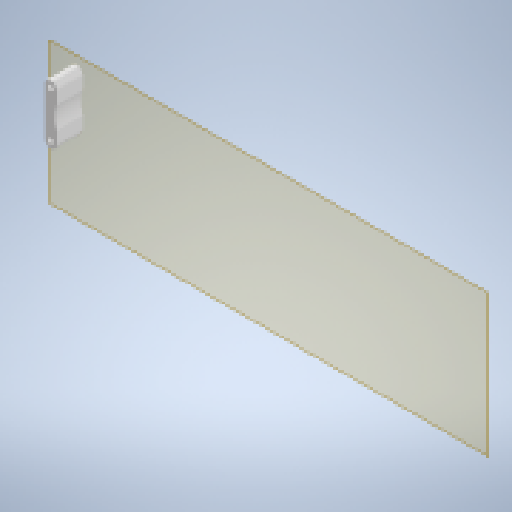
# Autodesk Inventor part: plate_washer_1
Saved by Autodesk Inventor 2024 (Build 280153000, 153)
## iProperties
Created: 2026-02-04
Part Number: plate_washer_1
Material: Generic
Document SubType Name: Modeling
Designer: SEMEN
Density: 1 g/cm^3
Appearance: Default
Author: SEMEN
Autodesk Inventor part; units mm, degrees
ref_plane "YZ Plane" through (0, 0, 0) normal (1, 0, 0) x (0, 1, 0)
ref_plane "XZ Plane" through (0, 0, 0) normal (0, 1, 0) x (-1, 0, 0)
ref_plane "XY Plane" through (0, 0, 0) normal (0, 0, 1) x (1, 0, 0)
ref_plane "Work Plane1" through (0, 0, 0) normal (0, 0, 1) x (1, 0, 0)
sketch "Sketch1" plane through (0, 0, 0) normal (0, 0, 1) x (1, 0, 0)
  circle A0 centre (-26, -15.5) radius 1.7 projected
  circle A1 centre (-26, 15.5) radius 1.7 projected
  arc A2 (-30.2, -15.5) -> (-21.8, -15.5) centre (-26, -15.5) ccw
  arc A3 (-21.8, 15.5) -> (-30.2, 15.5) centre (-26, 15.5) ccw
  arc A4 (-21.8, 7.3321) -> (-21.8, -7.3321) centre (0, 0) ccw
  line L0 (-21.8, -15.5) -> (-21.8, -7.3321)
  line L1 (-21.8, 7.3321) -> (-21.8, 15.5)
  line L2 (-30.2, -15.5) -> (-30.2, 15.5)
  line L3 (-26, -15.5) -> (-30.2, -15.5) construction
  dimension "d0" = 2.5
  dimension "d1" = 2.5
  dimension "d2" = 46
  constraints: 8 end point, 6 point on circle, 3 centre point, 3 tangent, 2 vertical, 1 coincident, 1 horizontal
  measures "d0" radial gap between concentric circles of A0 A2
  measures "d1" radial gap between concentric circles of A1 A3
  measures "d2" diameter of A4
extrude "Extrusion1" add sketch "Sketch1" along normal blind 18 contours A0 | A1 | L2 A3 L1 A4 L0 A2
hole "Hole1" at (-26, 15.5, 0) at (-26, -15.5, 0) direction (0, 0, 1) diameter 3.4 end through all clearance for "Countersunk Head GOST 12876-67" size "M3" standard "GOST"
body "Solid1"
